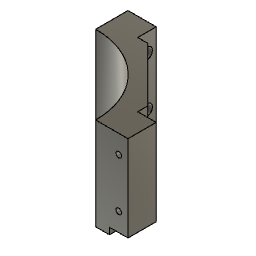
QuaterV2 v3 (Autodesk Fusion 360 design; units mm, degrees)
Autodesk Fusion 360 part; units mm, degrees
sketch "Body" plane through (0, 0, 0) normal (0, 0, 1) x (1, 0, 0)
  circle A0 centre (0, 0) radius 85
  line L0 (-100, -41.4214) -> (-41.4214, -100)
  line L1 (-41.4214, -100) -> (41.4214, -100)
  line L2 (41.4214, -100) -> (100, -41.4214)
  line L3 (100, -41.4214) -> (100, 41.4214)
  line L4 (100, 41.4214) -> (41.4214, 100)
  line L5 (41.4214, 100) -> (-41.4214, 100)
  line L6 (-41.4214, 100) -> (-100, 41.4214)
  line L7 (-100, 41.4214) -> (-100, -41.4214)
  line L8 (-30.5, -100) -> (30.5, -100)
  line L9 (30.5, -100) -> (30.5, -120)
  line L10 (30.5, -120) -> (-30.5, -120)
  line L11 (-30.5, -120) -> (-30.5, -100)
  line L12 (-30.5, 100) -> (30.5, 100)
  line L13 (30.5, 100) -> (30.5, 120)
  line L14 (30.5, 120) -> (-30.5, 120)
  line L15 (-30.5, 120) -> (-30.5, 100)
  line L16 (100, 30.5) -> (120, 30.5)
  line L17 (120, 30.5) -> (120, -30.5)
  line L18 (120, -30.5) -> (100, -30.5)
  line L19 (100, -30.5) -> (100, 30.5)
  line L20 (-100, 30.5) -> (-120, 30.5)
  line L21 (-120, 30.5) -> (-120, -30.5)
  line L22 (-120, -30.5) -> (-100, -30.5)
  line L23 (-100, -30.5) -> (-100, 30.5)
  line L24 (-120, 0) -> (120, 0)
  line L25 (0, 120) -> (0, -120)
  dimension "d1" = 170
  dimension "d2" = 100
  dimension "d4" = 61
  dimension "d5" = 20
  dimension "d7" = 61
  dimension "d8" = 20
  dimension "d10" = 61
  dimension "d11" = 20
  dimension "d13" = 20
  dimension "d14" = 61
  constraint coincident A0.centre origin
  constraint horizontal L8
  constraint vertical L9
  constraint horizontal L10
  constraint vertical L11
  constraint coincident L1 L8.start
  constraint horizontal L12
  constraint vertical L13
  constraint horizontal L14
  constraint vertical L15
  constraint coincident L5 L12.start
  constraint horizontal L16
  constraint vertical L17
  constraint horizontal L18
  constraint vertical L19
  constraint coincident L3 L16.start
  constraint horizontal L20
  constraint vertical L21
  constraint horizontal L22
  constraint vertical L23
  constraint coincident L7 L20.start
  constraint midpoint L21 L24.start
  constraint midpoint L17 L24.end
  constraint perpendicular L17 L24
  constraint midpoint L14 L25.start
  constraint midpoint L10 L25.end
  constraint perpendicular L10 L25
  measures "d1" diameter of A0
  measures "d2" distance of A0.centre L7
  measures "d4" distance of L8.start L8.end
  measures "d5" distance of L8.start L10.end
  measures "d7" distance of L12.start L12.end
  measures "d8" distance of L12.start L14.end
  measures "d10" distance of L16.start L18.end
  measures "d11" distance of L16.start L16.end
  measures "d13" distance of L20.start L20.end
  measures "d14" distance of L20.start L22.end
extrude "Extrude1" add sketch "Body" along normal blind 100 contours A0 L3 L4 L5 L12 L19 L24 L25 | L3 L16 L17 L19 L24 | L5 L12 L13 L14 L25
extrude "Extrude2" cut sketch "Body" along normal blind 7 contours L3 L16 L17 L19 L24 | L5 L12 L13 L14 L25
sketch "H_Circle" plane through (30.5, 0, 0) normal (1, 0, 0) x (0, 1, 0)
  line L0 (100, 7) -> (120, 7)
  line L1 (120, 7) -> (120, 100)
  line L2 (120, 100) -> (100, 100)
  line L3 (100, 100) -> (100, 7)
  line L4 (100, 100) -> (120, 100)
  line L5 (120, 100) -> (120, 7)
  line L6 (120, 7) -> (100, 7)
  line L7 (100, 7) -> (100, 100)
  line L8 (100, 100) -> (120, 100)
  line L9 (120, 100) -> (120, 80)
  line L10 (100, 80) -> (100, 100)
  line L11 (100, 7) -> (120, 7)
  line L12 (120, 7) -> (120, 27)
  line L13 (100, 27) -> (100, 7)
  circle A0 centre (110, 80) radius 6
  circle A1 centre (110, 80) radius 3
  circle A2 centre (110, 27) radius 6
  circle A3 centre (110, 27) radius 3
  dimension "d19" = 20
  dimension "d20" = 20
  dimension "d21" = 12
  dimension "d22" = 6
  dimension "d23" = 12
  dimension "d24" = 6
  constraint horizontal L4
  constraint vertical L5
  constraint horizontal L6
  constraint vertical L7
  constraint coincident L0.end L1.start
  constraint coincident L2.end L3.start
  constraint horizontal L8
  constraint vertical L9
  constraint vertical L10
  constraint coincident L5 L9.end
  constraint horizontal L11
  constraint vertical L12
  constraint vertical L13
  constraint concentric A0 A1
  constraint concentric A2 A3
  measures "d19" distance of L2.end L10.start
  measures "d20" distance of L0.start L13.start
  measures "d21" diameter of A0
  measures "d22" diameter of A1
  measures "d23" diameter of A2
  measures "d24" diameter of A3
extrude "Extrude3" cut sketch "H_Circle" against normal blind 70 contours A1 | A3
extrude "Extrude4" cut sketch "H_Circle" against normal blind 6 contours A0 | A2
sketch "H_Hex" plane through (0, 30.5, 0) normal (0, 1, 0) x (-1, 0, 0)
  line L0 (-120, 7) -> (-100, 7)
  line L1 (-100, 7) -> (-100, 100)
  line L2 (-100, 100) -> (-120, 100)
  line L3 (-120, 100) -> (-120, 7)
  line L4 (-120, 100) -> (-100, 100)
  line L5 (-100, 100) -> (-100, 7)
  line L6 (-100, 7) -> (-120, 7)
  line L7 (-120, 7) -> (-120, 100)
  line L8 (-120, 100) -> (-100, 100)
  line L9 (-100, 100) -> (-100, 80)
  line L10 (-120, 80) -> (-120, 100)
  line L11 (-120, 7) -> (-100, 7)
  line L12 (-100, 7) -> (-100, 27)
  line L13 (-120, 27) -> (-120, 7)
  circle A0 centre (-110, 80) radius 3
  circle A1 centre (-110, 27) radius 3
  line L14 (-115.5, 76.8246) -> (-110, 73.6491)
  line L15 (-110, 73.6491) -> (-104.5, 76.8246)
  line L16 (-104.5, 76.8246) -> (-104.5, 83.1754)
  line L17 (-104.5, 83.1754) -> (-110, 86.3509)
  line L18 (-110, 86.3509) -> (-115.5, 83.1754)
  line L19 (-115.5, 83.1754) -> (-115.5, 76.8246)
  line L20 (-115.5, 23.8246) -> (-110, 20.6491)
  line L21 (-110, 20.6491) -> (-104.5, 23.8246)
  line L22 (-104.5, 23.8246) -> (-104.5, 30.1754)
  line L23 (-104.5, 30.1754) -> (-110, 33.3509)
  line L24 (-110, 33.3509) -> (-115.5, 30.1754)
  line L25 (-115.5, 30.1754) -> (-115.5, 23.8246)
  point P0 (-110, 80)
  point P1 (-110, 27)
  dimension "d30" = 20
  dimension "d31" = 20
  dimension "d32" = 6
  dimension "d33" = 6
  dimension "d34" = 5.5
  dimension "d35" = 5.5
  constraint horizontal L4
  constraint vertical L5
  constraint horizontal L6
  constraint vertical L7
  constraint coincident L0.end L1.start
  constraint coincident L2.end L3.start
  constraint horizontal L8
  constraint vertical L9
  constraint vertical L10
  constraint horizontal L11
  constraint vertical L12
  constraint vertical L13
  constraint coincident P0 A0.centre
  constraint coincident P1 A1.centre
  measures "d30" distance of L0.start L0.end
  measures "d31" distance of L0.start L13.start
  measures "d32" diameter of A0
  measures "d33" diameter of A1
  measures "d34" distance of P0 L19
  measures "d35" distance of P1 L25
extrude "Extrude5" cut sketch "H_Hex" against normal blind 5 contours L14 L15 L16 L17 L18 L19 | L20 L21 L22 L23 L24 L25
extrude "Extrude6" cut 2 faces at (110.2225, 30.5, 80.9749) (109.2094, 30.5, 26.0676) along direction (0, -1, 0) blind 80
